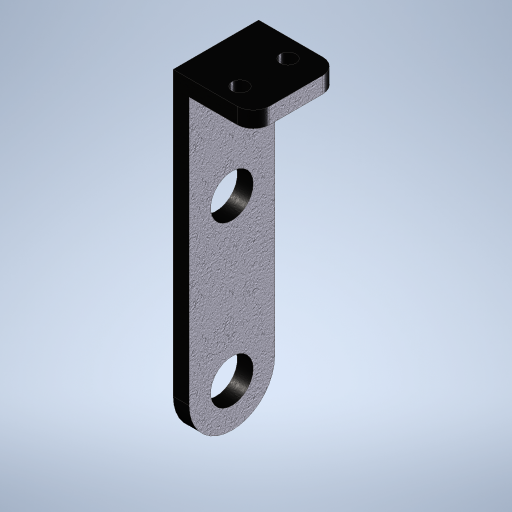
# Autodesk Inventor part: HUDSON-1-75
Saved by Autodesk Inventor 2024.2 (Build 282272000, 272)
## iProperties
Created: 2024-09-29
Part Number: HUDSON-1-75
Material: Generic
Document SubType Name: Modeling
Designer: melim
Density: 1 g/cm^3
Appearance: Galvanized
Author: melim
Autodesk Inventor part; units mm, degrees
ref_plane "YZ Plane" through (0, 0, 0) normal (1, 0, 0) x (0, 1, 0)
ref_plane "XZ Plane" through (0, 0, 0) normal (0, 1, 0) x (-1, 0, 0)
ref_plane "XY Plane" through (0, 0, 0) normal (0, 0, 1) x (1, 0, 0)
sketch "Sketch1" plane through (0, 0, 0) normal (0, 0, 1) x (1, 0, 0)
  line L0 (0, 0) -> (0, 61)
  line L1 (3, 0) -> (3, 58)
  line L2 (0, 0) -> (3, 0)
  line L3 (3, 58) -> (15, 58)
  line L4 (0, 61) -> (15, 61)
  line L5 (15, 58) -> (15, 61)
  point P0 (9, 61)
  dimension "d0" = 61
  dimension "d2" = 3
  dimension "d3" = 12
  dimension "d4" = 3
  constraints: 12 end point, 2 horizontal, 2 vertical, 1 parallel, 1 perpendicular, 1 point on line
  measures "d0" distance of L0.start L0.end
  measures "d2" distance between parallel lines of L0 L1
  measures "d3" distance of L1.end L3.end
  measures "d4" distance from line of point (9, 61) L3
extrude "Extrusion1" add sketch "Sketch1" along normal blind 16
fillet "Fillet1" radius 8 2 edges at (1.5, 0, 16) (1.5, 0, 0)
sketch "Sketch2" plane through (3, 58, 16) normal (1, 0, 0) x (0, 0, -1)
  arc A0 (0, -50) -> (16, -50) centre (8, -50) ccw construction
  line L0 (16, -50) -> (16, 0) construction
  line L1 (16, 0) -> (0, 0) construction
  line L2 (0, -50) -> (0, 0) construction
  line L3 (16, 3) -> (0, 3) projected
  point P0 (16, -58)
  point P1 (8, -20)
  dimension "d8" = 30
  dimension "d9" = 23
  dimension "d10" = 8
  dimension "d11" = 8
  measures "d8" distance of point (8, -20) point (8, -50)
  measures "d9" distance from line of L3 point (8, -20)
  measures "d10" distance from line of L2 point (8, -20)
  measures "d11" distance from line of L2 point (8, -50)
hole "Hole1" at (3, 8, 8) at (3, 38, 8) direction (-1, 0, 0) diameter 8 end through all
sketch "Sketch3" plane through (0, 61, 0) normal (0, 1, 0) x (1, 0, 0)
  line L0 (15, 0) -> (0, 0) projected
  line L1 (0, 0) -> (0, -16) projected
  line L2 (15, -16) -> (0, -16) projected
  line L3 (15, 0) -> (15, -16) projected
  point P0 (9, -12.5)
  point P1 (9, -3.5)
  point P2 (0, -8)
  dimension "d19" = 9
  dimension "d20" = 9
  dimension "d21" = 4.5
  constraints: 1 midpoint
  measures "d19" distance of point (9, -3.5) point (9, -12.5)
  measures "d20" distance from line of L1 point (9, -12.5)
  measures "d21" vertical distance of point (9, -3.5) point (0, -8)
hole "Hole2" at (9, 61, 12.5) at (9, 61, 3.5) direction (0, -1, 0) diameter 3 end through all
fillet "Fillet2" radius 3 2 edges at (15, 59.5, 16) (15, 59.5, 0)
body "Solid1"
